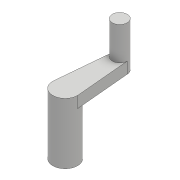
# Autodesk Inventor part: Part12
Saved by Autodesk Inventor 2017 (Build 210142000, 142)
## iProperties
Created: 2019-07-23
Part Number: Part12
Material: Generic
Document SubType Name: Modeling
Designer: Admin
Density: 1 g/cm^3
Appearance: Default
Mass: 46.9802 g
Surface Area: 103.74 cm^2
Volume: 46.9802 cm^3
Author: Admin
Autodesk Inventor part; units mm, degrees
ref_plane "YZ Plane" through (0, 0, 0) normal (1, 0, 0) x (0, 1, 0)
ref_plane "XZ Plane" through (0, 0, 0) normal (0, 1, 0) x (-1, 0, 0)
ref_plane "XY Plane" through (0, 0, 0) normal (0, 0, 1) x (1, 0, 0)
sketch "Sketch1" plane through (0, 0, 0) normal (0, 0, 1) x (1, 0, 0)
  circle A0 centre (0, 0) radius 12.5
  dimension "d0" = 25
  constraints: 1 centre point, 1 coincident
  measures "d0" diameter of A0
extrude "Extrusion1" add sketch "Sketch1" along normal blind 50
sketch "Sketch2" plane through (0, 0, 50) normal (0, 0, 1) x (1, 0, 0)
  circle A0 centre (0, 55.1215) radius 7.5
  line L0 (-7.5, 55.1215) -> (-12.5, 0)
  circle A1 centre (0, 0) radius 12.5 projected
  line L1 (7.5, 55.1215) -> (12.5, 0)
  dimension "d3" = 15
  constraints: 4 end point, 4 point on circle, 1 centre point
  measures "d3" diameter of A0
extrude "Extrusion2" add sketch "Sketch2" along normal blind 11.5 contours L1 A1 L0 A0 | L1 A1 L0
extrude "Extrusion3" add sketch "Sketch2" along normal blind 45 contours A0
body "Solid1"
